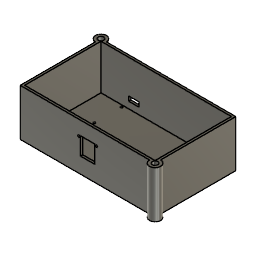
Modelo 3D de Taller de Diseñoen milimetros (Autodesk Fusion 360 design; units mm, degrees)
part number: 2026-05-21-14-10-05-150
Autodesk Fusion 360 part; units mm, degrees
note: some values were not read from the file. Set by a fixed rule: which sketch regions a step uses.
sketch "Boceto1" plane through (0, 0, 0) normal (0, 0, 1) x (1, 0, 0)
  line L0 (0, 0) -> (116.4, 0)
  line L1 (0, 0) -> (0, 68.1)
  line L2 (0, 0) -> (116.4, 0)
  line L3 (116.4, 0) -> (116.4, 68.1)
  line L4 (116.4, 68.1) -> (0, 68.1)
  line L5 (0, 68.1) -> (0, 0)
  dimension "d1" = 116.4
  dimension "d2" = 68.1
  constraint coincident L0.start L1.start
  constraint horizontal L0
  constraint perpendicular L0 L1
  constraint horizontal L2
  constraint vertical L3
  constraint horizontal L4
  constraint vertical L5
  measures "d1" distance of L0.start L0.end
  measures "d2" distance of L0.start L1.end
extrude "Extruir1" add sketch "Boceto1" along normal blind 39.9 makes body 1
shell "Vaciado1" thickness 2 outward yes removed faces 1 at (38.8, 22.7, 39.9) on bodies 1
hole "Agujero1" at (0, 8.975, 19.95) direction (-1, 0, 0) diameter 11.75 depth 2 tip angle 180 bodies 1
sketch "Boceto2" plane through (0, 0, 0) normal (0, 0, 1) x (1, 0, 0)
sketch "Boceto3" plane through (0, 0, 0) normal (0, 0, 1) x (1, 0, 0)
  line L0 (0, 0) -> (-9.1, 0)
  line L1 (0, 0) -> (0, 1.55)
  line L2 (0, 0) -> (-9.1, 0)
  line L3 (-9.1, 0) -> (-9.1, 1.55)
  line L4 (-9.1, 1.55) -> (0, 1.55)
  line L5 (0, 1.55) -> (0, 0)
  dimension "d11" = 9.1
  dimension "d12" = 1.55
  constraint coincident L0.start L1.start
  constraint horizontal L0
  constraint perpendicular L0 L1
  constraint horizontal L2
  constraint vertical L3
  constraint horizontal L4
  constraint vertical L5
  measures "d11" distance of L0.start L0.end
  measures "d12" distance of L0.start L1.end
sketch "Boceto4" plane through (0, 68.1, 0) normal (0, -1, 0) x (1, 0, 0)
  line L0 (0, 0) -> (116.4, 0)
  line L1 (116.4, 0) -> (116.4, 39.9)
  line L2 (116.4, 39.9) -> (0, 39.9)
  line L3 (0, 39.9) -> (0, 0)
sketch "Boceto5" plane through (0, 70.1, 0) normal (0, 1, 0) x (-1, 0, 0)
  line L0 (-118.4, -2) -> (2, -2)
  line L1 (2, -2) -> (2, 39.9)
  line L2 (2, 39.9) -> (-118.4, 39.9)
  line L3 (-118.4, 39.9) -> (-118.4, -2)
  line L4 (-24.8008, 9.9196) -> (-33.9008, 9.9196)
  line L5 (-33.9008, 9.9196) -> (-33.9008, 5.9196)
  line L6 (-33.9008, 5.9196) -> (-24.8008, 5.9196)
  line L7 (-24.8008, 5.9196) -> (-24.8008, 9.9196)
  line L8 (0, 0) -> (0, 9.92)
  line L9 (0, 17.6846) -> (-24.8, 17.6846)
  dimension "d15" = 9.1
  dimension "d16" = 4
  dimension "d17" = 9.92
  dimension "d18" = 24.8
  constraint horizontal L4
  constraint vertical L5
  constraint horizontal L6
  constraint vertical L7
  constraint coincident L8.start origin
  constraint perpendicular L2 L8
  constraint perpendicular L1 L9
  measures "d15" distance of L4.start L4.end
  measures "d16" distance of L4.start L6.end
  measures "d17" distance of L8.start L8.end
  measures "d18" distance of L9.start L9.end
extrude "Extruir3" cut sketch "Boceto5" against normal blind 2 contours L4 L5 L6 L7 bodies 1
sketch "Boceto6" plane through (0, -2, 0) normal (0, -1, 0) x (1, 0, 0)
  line L0 (-2, -2) -> (118.4, -2)
  line L1 (118.4, -2) -> (118.4, 39.9)
  line L2 (118.4, 39.9) -> (-2, 39.9)
  line L3 (-2, 39.9) -> (-2, -2)
  line L4 (0, 0) -> (0, 12.1)
  line L5 (51.7502, 27.8001) -> (64.6502, 27.8001)
  line L6 (64.6502, 27.8001) -> (64.6502, 12.1001)
  line L7 (64.6502, 12.1001) -> (51.7502, 12.1001)
  line L8 (51.7502, 12.1001) -> (51.7502, 27.8001)
  line L9 (0, 25.0106) -> (51.75, 25.0106)
  dimension "d22" = 12.1
  dimension "d23" = 12.9
  dimension "d24" = 15.7
  dimension "d25" = 51.75
  constraint coincident L4.start origin
  constraint parallel L3 L4
  constraint horizontal L5
  constraint vertical L6
  constraint horizontal L7
  constraint vertical L8
  constraint perpendicular L3 L9
  measures "d22" distance of L4.start L4.end
  measures "d23" distance of L5.start L5.end
  measures "d24" distance of L5.start L7.end
  measures "d25" distance of L9.start L9.end
extrude "Extruir4" cut sketch "Boceto6" against normal blind 2 contours L5 L6 L7 L8 bodies 1
sketch "Boceto7" plane through (0, 0, 0) normal (0, 0, 1) x (-1, 0, 0)
  line L0 (0, -68.1) -> (0, 0)
  line L1 (0, 0) -> (-116.4, 0)
  line L2 (-116.4, 0) -> (-116.4, -68.1)
  line L3 (-116.4, -68.1) -> (0, -68.1)
  line L4 (1.9318, 2.1365) -> (-118.3041, 2.1365)
  line L5 (-118.3041, 2.1365) -> (-118.3041, -69.8268)
  line L6 (-118.3041, -69.8268) -> (1.9318, -69.8268)
  line L7 (1.9318, -69.8268) -> (1.9318, 2.1365)
  constraint horizontal L4
  constraint vertical L5
  constraint horizontal L6
  constraint vertical L7
sketch "Boceto8" plane through (0, 0, 0) normal (0, 0, 1) x (1, 0, 0)
  line L0 (140.7037, 0) -> (20.3037, 0)
  line L1 (20.3037, 0) -> (20.3037, 72.1)
  line L2 (20.3037, 72.1) -> (140.7037, 72.1)
  line L3 (140.7037, 72.1) -> (140.7037, 0)
  dimension "d33" = 120.4
  dimension "d34" = 72.1
  constraint horizontal L0
  constraint vertical L1
  constraint horizontal L2
  constraint vertical L3
  measures "d33" distance of L0.start L0.end
  measures "d34" distance of L0.start L2.end
extrude "Extruir6" add sketch "Boceto8" along normal blind 2 separate body makes body 2
move_body "Desplazar6" bodies 2 to x (1, 0, 0) y (0, 1, 0) z (0, 0, 1) at (-20.3037, 0, 0)
move_body "Desplazar7" bodies 2 to x (1, 0, 0) y (0, 1, 0) z (0, 0, 1) at (0, 0, 68)
move_body "Desplazar8" bodies 2 to x (1, 0, 0) y (0, 1, 0) z (0, 0, 1) at (-2, 0, 0)
move_body "Desplazar9" bodies 2 to x (1, 0, 0) y (0, 1, 0) z (0, 0, 1) at (0, -2, 0)
sketch "Boceto9" plane through (-2, 0, 0) normal (-1, 0, 0) x (0, -1, 0)
  circle A0 centre (-8.975, 19.95) radius 5.875
  line L0 (-70.1, -2) -> (2, -2)
  line L1 (2, -2) -> (2, 39.9)
  line L2 (2, 39.9) -> (-70.1, 39.9)
  line L3 (-70.1, 39.9) -> (-70.1, -2)
  line L4 (-13.278, 23.95) -> (-4.672, 23.95)
  line L5 (-14.4991, 21.95) -> (-3.4509, 21.95)
  line L6 (-14.4991, 17.95) -> (-3.4509, 17.95)
  line L7 (-13.278, 15.95) -> (-4.672, 15.95)
  line L8 (-8.975, 19.95) -> (-0.4734, 19.95) construction
  line L9 (-14.85, 19.95) -> (-3.1, 19.95)
  dimension "d49" = 2
  dimension "d50" = 2
  dimension "d51" = 2
  dimension "d52" = 2
  constraint coincident A0 L4.start
  constraint coincident A0 L4.end
  constraint horizontal L4
  constraint coincident A0 L5.start
  constraint coincident A0 L5.end
  constraint parallel L4 L5
  constraint coincident A0 L6.start
  constraint coincident A0 L6.end
  constraint parallel L5 L6
  constraint coincident A0 L7.start
  constraint coincident A0 L7.end
  constraint parallel L4 L7
  constraint coincident A0.centre L8.start
  constraint parallel L4 L8
  constraint coincident A0 L9.start
  constraint coincident L8 L9.end
  constraint coincident A0 L9.end
  constraint parallel L8 L9
  measures "d49" distance of L5 L8
  measures "d50" distance of L6 L8
  measures "d51" distance of L4 L5
  measures "d52" distance of L6 L7
extrude "Extruir7" add sketch "Boceto9" against normal blind 2 contours A0 L5 L9 | A0 L6 L7 | A0 L4 bodies 1
sketch "Boceto10" plane through (0, -2, 0) normal (0, -1, 0) x (1, 0, 0)
  line L0 (64.6502, 27.8001) -> (64.6502, 12.1001)
  line L1 (64.6502, 12.1001) -> (51.7502, 12.1001)
  line L2 (51.7502, 12.1001) -> (51.7502, 27.8001)
  line L3 (51.7502, 27.8001) -> (64.6502, 27.8001)
  line L4 (-2, -2) -> (118.4, -2)
  line L5 (118.4, -2) -> (118.4, 39.9)
  line L6 (118.4, 39.9) -> (-2, 39.9)
  line L7 (-2, 39.9) -> (-2, -2)
sketch "Boceto11" plane through (0, 0, -2) normal (0, 0, -1) x (1, 0, 0)
  line L0 (-2, 2) -> (-2, -70.1)
  line L1 (-2, -70.1) -> (118.4, -70.1)
  line L2 (118.4, -70.1) -> (118.4, 2)
  line L3 (118.4, 2) -> (-2, 2)
  circle A0 centre (118.4, 2) radius 5
  dimension "d55" = 10
  constraint coincident L2.end L3.start
  measures "d55" diameter of A0
extrude "Extruir8" add sketch "Boceto11" against normal up to surface (41.9 mm away) contours L2 L3 A0 picked at (115.0853, 2.2484) bodies 1
sketch "Boceto12" plane through (0, 0, 39.9) normal (0, 0, 1) x (-1, 0, 0)
  line L0 (0, -68.1) -> (-116.4, -68.1)
  line L1 (-116.4, -68.1) -> (-116.4, 0)
  line L2 (-116.4, 0) -> (0, 0)
  line L3 (0, 0) -> (0, -68.1)
  line L4 (2, -70.1) -> (2, 2)
  line L5 (2, 2) -> (-113.4, 2)
  arc A0 (-113.4, 2) -> (-118.4, -3) centre (-118.4, 2) ccw
  line L6 (-118.4, -3) -> (-118.4, -70.1)
  line L7 (-118.4, -70.1) -> (2, -70.1)
  line L8 (-123.4, 2) -> (-118.4, 2)
  line L9 (-118.4, 2) -> (-118.4, -0.5)
  circle A1 centre (-118.4, 2) radius 2.5
  dimension "d58" = 2.5
  constraint coincident A0 L8.start
  constraint coincident A0.centre L8.end
  constraint perpendicular L1 L8
  constraint perpendicular L8 L9
  constraint coincident L9.end A1
  measures "d58" distance of A0.centre L9.end
extrude "Extruir9" cut sketch "Boceto12" against normal blind 4 contours L8 L9 A1 | L8 L9 A1 bodies 1
sketch "Boceto13" plane through (0, 0, -2) normal (0, 0, -1) x (1, 0, 0)
  line L0 (-2, 2) -> (-2, -70.1)
  line L1 (-2, -70.1) -> (118.4, -70.1)
  line L2 (118.4, -70.1) -> (118.4, -3)
  arc A0 (118.4, -3) -> (113.4, 2) centre (118.4, 2) ccw
  line L3 (113.4, 2) -> (-2, 2)
  circle A1 centre (-2, -70.1) radius 5
  dimension "d61" = 10
  constraint coincident L0.end L1.start
  measures "d61" diameter of A1
extrude "Extruir10" add sketch "Boceto13" against normal blind 41.9 contours L0 L1 A1 picked at (1.2435, -70.8284) bodies 1
sketch "Boceto14" plane through (0, 0, 39.9) normal (0, 0, 1) x (-1, 0, 0)
  circle A0 centre (-118.4, 2) radius 2.5
  line L0 (0, -68.1) -> (-116.4, -68.1)
  line L1 (-116.4, -68.1) -> (-116.4, 0)
  line L2 (-116.4, 0) -> (0, 0)
  line L3 (0, 0) -> (0, -68.1)
  line L4 (2, -65.1) -> (2, 2)
  line L5 (2, 2) -> (-113.4, 2)
  arc A1 (-113.4, 2) -> (-118.4, -3) centre (-118.4, 2) ccw
  line L6 (-118.4, -3) -> (-118.4, -70.1)
  line L7 (-118.4, -70.1) -> (-3, -70.1)
  arc A2 (-3, -70.1) -> (2, -65.1) centre (2, -70.1) ccw
  line L8 (7, -70.1) -> (2, -70.1)
  circle A3 centre (2, -70.1) radius 2.5
  dimension "d64" = 5
  dimension "d65" = 5
  constraint coincident A2 L8.start
  constraint parallel L0 L8
  constraint concentric A2 A3
  measures "d64" distance of L8.start A2.centre
  measures "d65" diameter of A3
extrude "Extruir11" cut sketch "Boceto14" against normal blind 4 contours A3 bodies 1
sketch "Boceto15" plane through (0, 0, 70) normal (0, 0, 1) x (-1, 0, 0)
  line L0 (-118.4, -70.1) -> (2, -70.1)
  line L1 (2, -70.1) -> (2, 2)
  line L2 (2, 2) -> (-118.4, 2)
  line L3 (-118.4, 2) -> (-118.4, -70.1)
sketch "Boceto16" plane through (0, 0, 70) normal (0, 0, 1) x (-1, 0, 0)
  line L0 (1.998, -70.0962) -> (6.998, -70.0962)
  line L1 (-118.3904, 1.9889) -> (-123.3904, 1.9889)
  circle A0 centre (-118.3904, 1.9889) radius 5
  circle A1 centre (1.998, -70.0962) radius 5
  dimension "d68" = 5
  dimension "d69" = 5
  constraint horizontal L0
  constraint horizontal L1
  constraint coincident L1.start A0.centre
  constraint coincident L1.end A0
  constraint coincident L0.start A1.centre
  constraint coincident L0.end A1
  measures "d68" distance of L0.start L0.end
  measures "d69" distance of L1.start L1.end
extrude "Extruir12" add sketch "Boceto16" against normal blind 2 contours A1 bodies 2
extrude "Extruir13" add sketch "Boceto16" against normal blind 2 contours A0 bodies 2
sketch "Boceto17" plane through (0, -2, 0) normal (0, -1, 0) x (1, 0, 0)
hole "Agujero2" at (118.3904, -1.9889, 70) direction (0, 0, -1) diameter 3 depth 10 tip angle 118 bodies 2
hole "Agujero3" at (-2, 70.1, 70) direction (0, 0, -1) diameter 3 depth 5 tip angle 118 bodies 2
sketch "Boceto18" plane through (0, 0, 0) normal (0, 0, 1) x (-1, 0, 0)
  line L0 (0, -68.1) -> (0, 0)
  line L1 (0, 0) -> (-116.4, 0)
  line L2 (-116.4, 0) -> (-116.4, -68.1)
  line L3 (-116.4, -68.1) -> (0, -68.1)
  line L4 (-116.4, -67.1002) -> (-115.4, -67.1002)
  line L5 (-115.3999, -68.1) -> (-115.3999, -67.1)
  line L6 (-115.4, -67.1002) -> (-114.3087, -65.7967)
  circle A0 centre (-114.8543, -66.4483) radius 0.8499
  line L7 (-114.8543, -66.4483) -> (-115.7042, -66.4483)
  line L8 (-114.8543, -66.4483) -> (-114.0044, -66.4483)
  line L9 (-115.7042, -66.4483) -> (-18.9742, -66.4483)
  line L10 (-114.0044, -66.4483) -> (-20.6744, -66.4483)
  circle A1 centre (-19.8243, -66.4483) radius 0.8501
  line L11 (-19.8243, -66.4483) -> (-19.8243, -67.2984)
  line L12 (-19.8243, -66.4483) -> (-19.8243, -65.5982)
  line L13 (-19.8243, -67.2984) -> (-19.8243, -41.0484)
  line L14 (-19.8243, -65.5982) -> (-19.8243, -42.3182)
  circle A2 centre (-19.8243, -41.4682) radius 0.85
  line L15 (-19.8243, -41.4682) -> (-18.9743, -41.4682)
  line L16 (-19.8243, -41.4682) -> (-20.6743, -41.4682)
  line L17 (-18.9743, -41.4682) -> (-115.7043, -41.4682)
  line L18 (-20.6743, -41.4682) -> (-114.0043, -41.4682)
  circle A3 centre (-114.8543, -41.4682) radius 0.85
  dimension "d80" = 1
  dimension "d81" = 1
  dimension "d82" = 1.7
  dimension "d83" = 96.73
  dimension "d84" = 93.33
  dimension "d85" = 26.25
  dimension "d86" = 23.28
  dimension "d87" = 1.7
  dimension "d88" = 96.73
  dimension "d89" = 93.33
  constraint coincident L2 L4.start
  constraint perpendicular L2 L4
  constraint coincident L3 L5.start
  constraint perpendicular L3 L5
  constraint coincident L6.end A0
  constraint coincident L5.end A0
  constraint coincident A0.centre L7.start
  constraint coincident A0 L7.end
  constraint horizontal L7
  constraint coincident A0 L8.end
  constraint parallel L7 L8
  constraint parallel L8 L9
  constraint parallel L9 L10
  constraint coincident L9.end A1
  constraint coincident L10.end A1
  constraint coincident A1.centre L11.start
  constraint coincident A1 L11.end
  constraint perpendicular L9 L11
  constraint coincident A1 L12.end
  constraint perpendicular L9 L12
  constraint parallel L12 L13
  constraint parallel L13 L14
  constraint coincident L14.end A2
  constraint coincident A2.centre L15.start
  constraint coincident A2 L15.end
  constraint perpendicular L13 L15
  constraint coincident A2 L16.end
  constraint perpendicular L13 L16
  constraint parallel L15 L17
  constraint parallel L17 L18
  constraint coincident L18.end A3
  constraint coincident L17.end A3
  measures "d80" distance of L4.start L4.end
  measures "d81" distance of L5.start L5.end
  measures "d82" distance of L4.end L6.end
  measures "d83" distance of L7.end L9.end
  measures "d84" distance of L8.end L10.end
  measures "d85" distance of L11.end L13.end
  measures "d86" distance of L12.end L14.end
  measures "d87" diameter of A2
  measures "d88" distance of L15.end L17.end
  measures "d89" distance of L16.end L18.end
sketch "Boceto19" plane through (0, 0, 0) normal (1, 0, 0) x (0, 1, 0)
  circle A0 centre (9.004, 19.9495) radius 5.8433
sketch "Boceto20" plane through (0, 0, 0) normal (1, 0, 0) x (0, 1, 0)
  arc A0 (3.1, 19.95) -> (3.4509, 17.95) centre (8.975, 19.95) ccw
  line L0 (3.1, 19.95) -> (14.85, 19.95)
  arc A1 (14.4991, 17.95) -> (14.85, 19.95) centre (8.975, 19.95) ccw
  line L1 (14.4991, 17.95) -> (3.4509, 17.95)
  arc A2 (4.672, 23.95) -> (3.4509, 21.95) centre (8.975, 19.95) ccw
  line L2 (4.672, 23.95) -> (13.278, 23.95)
  arc A3 (14.4991, 21.95) -> (13.278, 23.95) centre (8.975, 19.95) ccw
  line L3 (14.4991, 21.95) -> (3.4509, 21.95)
  line L4 (4.672, 15.95) -> (13.278, 15.95)
  arc A4 (4.672, 15.95) -> (13.278, 15.95) centre (8.975, 19.95) ccw
  line L5 (0, 0) -> (68.1, 0)
  line L6 (68.1, 0) -> (68.1, 39.9)
  line L7 (68.1, 39.9) -> (0, 39.9)
  line L8 (0, 39.9) -> (0, 0)
  line L9 (0.7009, 25.9425) -> (0.7009, 14.1225)
  line L10 (1.0476, 24.2926) -> (1.067, 25.1424)
  line L11 (1.0476, 24.2926) -> (1.0424, 23.4426)
  line L12 (1.0424, 23.4426) -> (1.0424, 14.9126)
  line L13 (8.975, 25.7927) -> (8.975, 14.075)
  line L14 (8.975, 19.95) -> (8.975, 14.075)
  line L15 (0.7009, 15.691) -> (0.7009, 19.951)
  line L16 (0.7009, 19.951) -> (8.975, 19.95)
  dimension "d90" = 11.82
  dimension "d91" = 0.85
  dimension "d92" = 0.85
  dimension "d93" = 8.53
  dimension "d95" = 4.26
  constraint perpendicular L2 L9
  constraint parallel L9 L12
  constraint midpoint A4 L13.end
  constraint perpendicular L1 L13
  constraint coincident A0.centre A1.centre
  constraint coincident L9 L15.start
  constraint parallel L12 L15
  measures "d90" distance of L9.start L9.end
  measures "d91" distance of L10.start L10.end
  measures "d92" distance of L10.start L11.end
  measures "d93" distance of L11.end L12.end
  measures "d95" distance of L15.start L15.end
sketch "Boceto21" plane through (0, 0, 0) normal (1, 0, 0) x (0, 1, 0)
sketch "Boceto22" plane through (0, 0, -2) normal (0, 0, -1) x (1, 0, 0)
  line L0 (3, -70.1) -> (118.4, -70.1)
  line L1 (118.4, -70.1) -> (118.4, -3)
  arc A0 (118.4, -3) -> (113.4, 2) centre (118.4, 2) ccw
  line L2 (113.4, 2) -> (-2, 2)
  line L3 (-2, 2) -> (-2, -65.1)
  arc A1 (-2, -65.1) -> (3, -70.1) centre (-2, -70.1) ccw
sketch "Boceto23" plane through (0, 0, 0) normal (0, 0, 1) x (-1, 0, 0)
  line L0 (-116.4004, -67.0986) -> (-115.4004, -67.0986)
  line L1 (-115.4005, -68.0985) -> (-115.4005, -67.0985)
  circle A0 centre (-114.7042, -66.416) radius 0.975
  line L2 (-114.7042, -66.416) -> (-113.7292, -66.416)
  line L3 (-114.7042, -66.416) -> (-115.6792, -66.416)
  line L4 (-113.7292, -66.416) -> (-21.1792, -66.416)
  circle A1 centre (-20.2042, -66.416) radius 0.975
  line L5 (-20.2042, -66.416) -> (-20.2042, -65.441)
  line L6 (-20.2042, -66.416) -> (-20.2042, -67.391)
  line L7 (-20.2042, -65.441) -> (-20.2042, -42.871)
  circle A2 centre (-20.2042, -41.896) radius 0.975
  line L8 (-114.7042, -66.416) -> (-114.7042, -65.441)
  line L9 (-114.7042, -66.416) -> (-114.7042, -67.391)
  line L10 (-114.7042, -65.441) -> (-114.7042, -42.871)
  circle A3 centre (-114.7042, -41.896) radius 0.975
  dimension "d97" = 1
  dimension "d98" = 1
  dimension "d99" = 1.95
  dimension "d100" = 92.55
  dimension "d101" = 1.95
  dimension "d102" = 22.57
  dimension "d103" = 1.95
  dimension "d104" = 22.57
  dimension "d105" = 1.95
  constraint horizontal L0
  constraint vertical L1
  constraint coincident L0.end A0
  constraint coincident A0.centre L2.start
  constraint coincident A0 L2.end
  constraint coincident A0 L3.end
  constraint parallel L2 L4
  constraint coincident L4.end A1
  constraint coincident A1.centre L5.start
  constraint coincident A1 L5.end
  constraint vertical L5
  constraint coincident A1 L6.end
  constraint parallel L5 L6
  constraint parallel L5 L7
  constraint coincident L7.end A2
  constraint coincident A0 L8.end
  constraint perpendicular L3 L8
  constraint coincident A0 L9.end
  constraint perpendicular L3 L9
  constraint parallel L8 L10
  constraint coincident L10.end A3
  measures "d97" distance of L0.start L0.end
  measures "d98" distance of L1.start L1.end
  measures "d99" diameter of A0
  measures "d100" distance of L2.end L4.end
  measures "d101" diameter of A1
  measures "d102" distance of L5.end L7.end
  measures "d103" diameter of A2
  measures "d104" distance of L8.end L10.end
  measures "d105" diameter of A3
sketch "Boceto24" plane through (0, 0, 0) normal (0, 1, 0) x (-1, 0, 0)
  line L0 (-64.6502, 12.1001) -> (-64.6502, 27.8001)
  line L1 (-64.6502, 27.8001) -> (-51.7502, 27.8001)
  line L2 (-51.7502, 27.8001) -> (-51.7502, 12.1001)
  line L3 (-51.7502, 12.1001) -> (-64.6502, 12.1001)
  line L4 (-116.4, 0) -> (0, 0)
  line L5 (0, 0) -> (0, 39.9)
  line L6 (0, 39.9) -> (-116.4, 39.9)
  line L7 (-116.4, 39.9) -> (-116.4, 0)
  line L8 (-51.7502, 27.8001) -> (-48.3502, 27.8001)
  line L9 (-48.3502, 27.8001) -> (-48.3502, 25.8001)
  circle A0 centre (-50.7752, 26.8251) radius 0.975
  line L10 (-64.6502, 27.8001) -> (-68.0502, 27.8001)
  circle A1 centre (-65.6252, 26.8251) radius 0.975
  dimension "d106" = 3.4
  dimension "d107" = 2
  dimension "d108" = 0.975
  dimension "d109" = 3.4
  dimension "d110" = 0.975
  constraint coincident L1.end L2.start
  constraint perpendicular L2 L8
  constraint perpendicular L8 L9
  constraint tangent L8 A0
  constraint tangent L2 A0
  constraint coincident L0.end L1.start
  constraint perpendicular L0 L10
  constraint tangent L10 A1
  constraint tangent L0 A1
  measures "d106" distance of L1.end L8.end
  measures "d107" distance of L8.end L9.end
  measures "d108" radius of A0
  measures "d109" distance of L0.end L10.end
  measures "d110" radius of A1
sketch "Boceto25" plane through (0, 0, 0) normal (0, 0, 1) x (-1, 0, 0)
  line L0 (0, -68.1) -> (0, 0)
  line L1 (0, 0) -> (-116.4, 0)
  line L2 (-116.4, 0) -> (-116.4, -68.1)
  line L3 (-116.4, -68.1) -> (0, -68.1)
extrude "Extruir14" cut sketch "Boceto23" along normal blind 0 and the other way blind 3 contours A3 bodies 1
extrude "Extruir15" cut sketch "Boceto23" along normal blind 0 and the other way blind 3 contours A2 bodies 1
sketch "Boceto26" plane through (0, 0, 0) normal (0, 0, 1) x (-1, 0, 0)
  circle A0 centre (-20.2042, -41.896) radius 0.975
  line L0 (-20.2042, -41.896) -> (-20.2042, -40.9214)
  line L1 (-20.2042, -40.9214) -> (-20.2042, -38.4214)
  line L2 (-20.2042, -38.4214) -> (-20.2042, -36.4214)
  circle A1 centre (-20.2042, -37.4464) radius 0.975
  line L3 (-20.2042, -36.4714) -> (-20.2042, -14.6714)
  circle A2 centre (-20.2042, -13.6964) radius 0.975
  line L4 (-20.2042, -13.6964) -> (-21.1792, -13.6964)
  line L5 (-20.2042, -13.6964) -> (-19.2292, -13.6964)
  line L6 (-21.1792, -13.6964) -> (-70.5592, -13.6964)
  circle A3 centre (-71.5342, -13.6964) radius 0.975
  line L7 (-20.2042, -37.4464) -> (-21.1792, -37.4464)
  line L8 (-21.1792, -37.4464) -> (-70.5592, -37.4464)
  circle A4 centre (-71.5342, -37.4464) radius 0.975
  dimension "d119" = 2.5
  dimension "d120" = 2
  dimension "d121" = 1.95
  dimension "d122" = 21.8
  dimension "d123" = 1.95
  dimension "d124" = 49.38
  dimension "d125" = 1.95
  dimension "d126" = 49.38
  dimension "d127" = 1.95
  constraint coincident A0.centre L0.start
  constraint vertical L0
  constraint parallel L0 L1
  constraint parallel L1 L2
  constraint coincident L1.end A1
  constraint coincident L2 L3.start
  constraint coincident A1 L3.start
  constraint parallel L2 L3
  constraint coincident L3.end A2
  constraint coincident A2.centre L4.start
  constraint coincident A2 L4.end
  constraint horizontal L4
  constraint coincident A2 L5.end
  constraint parallel L4 L5
  constraint parallel L4 L6
  constraint coincident L6.end A3
  constraint coincident A1.centre L7.start
  constraint coincident A1 L7.end
  constraint perpendicular L2 L7
  constraint perpendicular L2 L8
  constraint coincident L8.end A4
  measures "d119" distance of L0.end L1.end
  measures "d120" distance of L1.end L2.end
  measures "d121" diameter of A1
  measures "d122" distance of L3.start L3.end
  measures "d123" diameter of A2
  measures "d124" distance of L4.end L6.end
  measures "d125" diameter of A3
  measures "d126" distance of L7.end L8.end
  measures "d127" diameter of A4
extrude "Extruir16" cut sketch "Boceto26" against normal blind 3 contours L2 A1 L7 | L2 A1 | L2 A1 L7 bodies 1
extrude "Extruir17" cut sketch "Boceto26" against normal blind 3 contours A4 bodies 1
extrude "Extruir18" cut sketch "Boceto26" against normal blind 3 contours A3 bodies 1
extrude "Extruir19" cut sketch "Boceto26" along normal blind -3 and the other way blind 0 contours A2 L4 L5 | A2 L4 L5 bodies 1
extrude "Extruir20" cut sketch "Boceto23" along normal blind -3 and the other way blind 0 contours A0 L2 L8 | A0 L2 L9 | A0 L3 L8 | A0 L3 L9 bodies 1
extrude "Extruir21" cut sketch "Boceto23" along normal blind -3000 and the other way blind 0 contours A1 L5 L6 | A1 L5 L6 bodies 1
extrude "Extruir22" add 1 faces at (64.6502, -1.3333, 22.5668) along direction (-1, 0, 0) blind 0.05 on bodies 1 bodies 1
extrude "Extruir23" add 1 faces at (51.7502, -1.3333, 17.3334) along direction (1, 0, 0) blind 0.05 on bodies 1 bodies 1
extrude "Extruir24" add 1 faces at (64.6002, -1.3333, 22.5668) along direction (-1, 0, 0) blind 0.05 on bodies 1 bodies 1
extrude "Extruir25" add 1 faces at (51.8002, -1.3333, 17.3334) along direction (1, 0, 0) blind 0.05 on bodies 1 bodies 1
sketch "Boceto27" plane through (0, 0, 0) normal (0, 1, 0) x (-1, 0, 0)
  line L0 (-64.5502, 27.8001) -> (-51.8502, 27.8001)
  line L1 (-51.8502, 27.8001) -> (-51.8502, 12.1001)
  line L2 (-51.8502, 12.1001) -> (-64.5502, 12.1001)
  line L3 (-64.5502, 12.1001) -> (-64.5502, 27.8001)
  line L4 (-116.4, 0) -> (0, 0)
  line L5 (0, 0) -> (0, 39.9)
  line L6 (0, 39.9) -> (-116.4, 39.9)
  line L7 (-116.4, 39.9) -> (-116.4, 0)
  line L8 (-51.8502, 27.8001) -> (-51.3002, 27.8001)
  line L9 (-64.5502, 27.8001) -> (-65.1002, 27.8001)
  line L10 (-51.3002, 27.8001) -> (-51.3002, 25.8501)
  line L11 (-65.1002, 27.8001) -> (-65.1002, 25.8501)
  circle A0 centre (-50.3252, 26.8251) radius 0.975
  circle A1 centre (-66.0752, 26.8251) radius 0.975
  dimension "d154" = 0.55
  dimension "d155" = 0.55
  dimension "d156" = 1.95
  dimension "d157" = 1.95
  dimension "d158" = 1.95
  dimension "d159" = 1.95
  constraint coincident L0.end L1.start
  constraint perpendicular L1 L8
  constraint coincident L0.start L3.end
  constraint perpendicular L3 L9
  constraint perpendicular L8 L10
  constraint perpendicular L9 L11
  measures "d154" distance of L0.end L8.end
  measures "d155" distance of L0.start L9.end
  measures "d156" distance of L8.end L10.end
  measures "d157" distance of L9.end L11.end
  measures "d158" diameter of A0
  measures "d159" diameter of A1
extrude "Extruir26" cut sketch "Boceto27" along normal blind -3 and the other way blind 0 contours A1 bodies 1
extrude "Extruir27" cut sketch "Boceto27" along normal blind -3 and the other way blind 0 contours A0 bodies 1
sketch "Boceto28" plane through (0, 0, 0) normal (1, 0, 0) x (0, 1, 0)
  arc A0 (3.1, 19.95) -> (3.4509, 17.95) centre (8.975, 19.95) ccw
  line L0 (3.1, 19.95) -> (14.85, 19.95)
  arc A1 (14.4991, 17.95) -> (14.85, 19.95) centre (8.975, 19.95) ccw
  line L1 (14.4991, 17.95) -> (3.4509, 17.95)
  arc A2 (4.672, 23.95) -> (3.4509, 21.95) centre (8.975, 19.95) ccw
  line L2 (4.672, 23.95) -> (13.278, 23.95)
  arc A3 (14.4991, 21.95) -> (13.278, 23.95) centre (8.975, 19.95) ccw
  line L3 (14.4991, 21.95) -> (3.4509, 21.95)
  line L4 (4.672, 15.95) -> (13.278, 15.95)
  arc A4 (4.672, 15.95) -> (13.278, 15.95) centre (8.975, 19.95) ccw
  line L5 (0, 0) -> (68.1, 0)
  line L6 (68.1, 0) -> (68.1, 39.9)
  line L7 (68.1, 39.9) -> (0, 39.9)
  line L8 (0, 39.9) -> (0, 0)
  line L9 (8.975, 14.075) -> (8.975, 25.675)
  line L10 (8.975, 19.875) -> (0, 19.875)
  line L11 (8.975, 25.675) -> (0, 25.675)
  line L12 (8.975, 14.075) -> (0, 14.075)
  line L13 (0, 19.875) -> (1.55, 19.875)
  line L14 (1.55, 19.875) -> (1.55, 16.375)
  line L15 (1.55, 19.875) -> (1.55, 23.375)
  line L16 (1.55, 16.375) -> (1.55, 15.825)
  line L17 (1.55, 23.375) -> (1.55, 23.925)
  circle A5 centre (1.55, 24.9) radius 0.975
  circle A6 centre (1.55, 14.85) radius 0.975
  dimension "d168" = 11.6
  dimension "d169" = 1.55
  dimension "d170" = 3.5
  dimension "d171" = 3.5
  dimension "d172" = 0.55
  dimension "d173" = 0.55
  dimension "d174" = 1.95
  dimension "d175" = 1.95
  constraint midpoint A4 L9.start
  constraint vertical L9
  constraint midpoint L9 L10.start
  constraint coincident L8 L10.end
  constraint perpendicular L8 L10
  constraint coincident L8 L11.end
  constraint perpendicular L8 L11
  constraint coincident L8 L12.end
  constraint tangent A4 L12
  constraint perpendicular L8 L12
  constraint perpendicular L8 L13
  constraint perpendicular L10 L14
  constraint perpendicular L13 L15
  constraint parallel L14 L16
  constraint parallel L15 L17
  constraint coincident L17.end A5
  constraint coincident L16.end A6
  measures "d168" distance of L9.start L9.end
  measures "d169" distance of L10.end L13.end
  measures "d170" distance of L13.end L14.end
  measures "d171" distance of L13.end L15.end
  measures "d172" distance of L14.end L16.end
  measures "d173" distance of L15.end L17.end
  measures "d174" diameter of A5
  measures "d175" diameter of A6
extrude "Extruir28" cut sketch "Boceto28" along normal blind -3 and the other way blind 0 contours L11 A5 | L11 A5 bodies 1
extrude "Extruir29" cut sketch "Boceto28" along normal blind -3 and the other way blind 0 contours L12 A6 | L12 A6 bodies 1
hidden bodies 2
equation "d50 = d49"
equation "d51 = d49"
